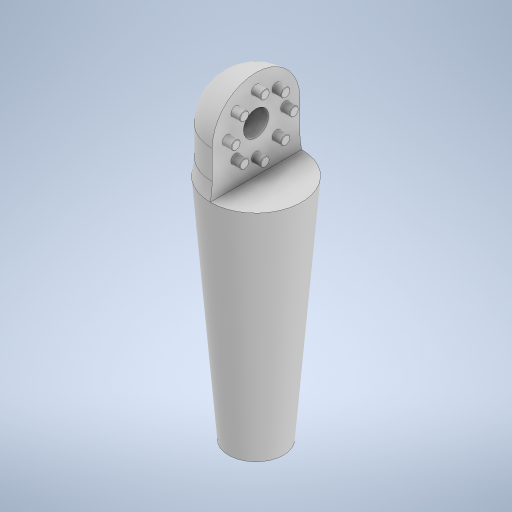
# Autodesk Inventor part: Connector_Male_V4
Saved by Autodesk Inventor 2024 (Build 280153000, 153)
## iProperties
Created: 2025-01-29
Part Number: Connector_Male_V4
Material: Generic
Document SubType Name: Modeling
Designer: b_arm
Density: 1 g/cm^3
Appearance: Default
Author: b_arm
## iProperties of the stored document CONNECT MALE V2_3DPrint.ipt
Created: 2025-02-18
Part Number: CONNECT MALE V2_3DPrint
Material: Generic
Document SubType Name: Modeling
Designer: b_arm
Density: 1 g/cm^3
Appearance: Default
Author: b_arm
Autodesk Inventor part; units mm, degrees
ref_plane "YZ Plane" through (0, 0, 0) normal (1, 0, 0) x (0, 1, 0)
ref_plane "XY Plane" through (0, 0, 0) normal (0, 0, 1) x (1, 0, 0)
sketch "Sketch1" plane through (0, 0, 0) normal (0, 1, 0) x (-1, 0, 0)
  circle A0 centre (0, 0) radius 7.62
  dimension "d0" = 15.24
  constraints: 1 centre point, 1 coincident
  measures "d0" diameter of A0
ref_plane "Work Plane1" through (0, 63.5, 0) normal (0, 1, 0) x (-1, 0, 0)
sketch "Sketch2" plane through (0, 63.5, 0) normal (0, 1, 0) x (-1, 0, 0)
  circle A0 centre (0, 0) radius 12.7
  dimension "d3" = 25.4
  constraints: 1 centre point, 1 coincident
  measures "d3" diameter of A0
loft "Loft1" add profiles "Sketch1", "Sketch2"
sketch "Sketch3" plane through (0, 63.5, 0) normal (0, 1, 0) x (1, 0, 0)
  arc A0 (0, 12.7) -> (0, -12.7) centre (0, 0) ccw
  line L0 (0, -12.7) -> (0, 12.7)
  constraints: 2 end point, 2 point on circle, 1 centre point, 1 coincident, 1 vertical
extrude "Extrusion1" add sketch "Sketch3" along normal blind 25.4
sketch "Sketch4" plane through (0, 63.5, 12.7) normal (1, 0, 0) x (0, 0, -1)
  line L0 (0, 25.4) -> (25.4, 25.4)
  line L1 (0, 0) -> (0, 25.4)
  line L2 (0, 12.7) -> (25.4, 12.7)
  line L3 (25.4, 0) -> (25.4, 25.4)
  circle A0 centre (12.7, 20.79625) radius 1.27
  line L4 (12.7, 12.7) -> (12.7, 15.916162)
  circle A1 centre (6.975087, 18.424913) radius 1.27
  circle A2 centre (4.60375, 12.7) radius 1.27
  circle A3 centre (6.975087, 6.975087) radius 1.27
  circle A4 centre (12.7, 4.60375) radius 1.27
  circle A5 centre (18.424913, 6.975087) radius 1.27
  circle A6 centre (20.79625, 12.7) radius 1.27
  circle A7 centre (18.424913, 18.424913) radius 1.27
  point P0 (12.7, -63.5)
  dimension "d12" = 2.54
  dimension "d15" = 360
  constraints: 8 centre point, 4 end point, 3 midpoint, 1 vertical, 17 other
  measures "d12" diameter of A0
extrude "Extrusion2" add sketch "Sketch4" along normal blind 2.54 contours A2 L2 | L2 A2 | A6 L2 | L2 A6 | A0 | A1 | A3 | A4 | A5 | A7
fillet "Fillet1" radius 0.127 8 edges at (2.54, 84.2963, 1.27) (2.54, 81.9249, -4.4549) (2.54, 76.2, -6.8262) (2.54, 70.4751, -4.4549) (2.54, 68.1038, 1.27) (2.54, 81.9249, 6.9949) (2.54, 76.2, 9.3663) (2.54, 70.4751, 6.9949)
fillet "Fillet2" radius 12.7 1 edges at (-12.7, 88.9, 0)
sketch "Sketch5" plane through (0, 63.5, 12.7) normal (1, 0, 0) x (0, 0, -1)
  circle A0 centre (12.7, 12.7) radius 3.49885
  point P0 (12.7, -63.5)
  dimension "d21" = 6.9977
  constraints: 1 centre point
  measures "d21" diameter of A0
extrude "Extrusion3" cut sketch "Sketch5" against normal blind 7.62
sketch "Sketch6" plane through (0, 0, 0) normal (0, -1, 0) x (1, 0, 0)
  circle A0 centre (0, 0) radius 5.24002
  dimension "d24" = 10.48004
  constraints: 1 centre point, 1 coincident
  measures "d24" diameter of A0
extrude "Extrusion4" cut sketch "Sketch6" against normal blind 50.8
thicken "Thicken1" operation cut thickness 0.508 both sides no extend neighbours no toward (0.9299564, -0.1318964, 0.3431973) faces at (-11.810448, 77.875171, -4.358605) (-0.000029, 88.9, 0.000017) (-12.7, 71.966733, 0)
fillet "Fillet3" radius 22.225 1 edges at (-12.192, 63.5, 0)
body "Solid1"
